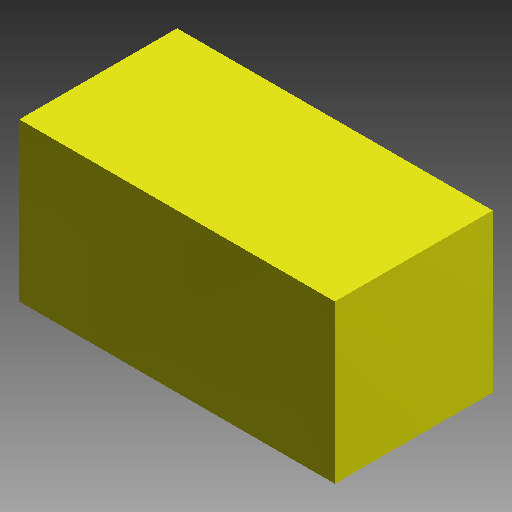
# Autodesk Inventor part: 1K
Saved by Autodesk Inventor 2018.2 (Build 222227000, 227)
## iProperties
Part Number: 1K
Material: Generic
Document SubType Name: Modeling
Designer: autocad
Appearance: R0603, 1K
Author: autocad
Autodesk Inventor part; units mm, degrees
ref_plane "YZ Plane" through (0, 0, 0) normal (1, 0, 0) x (0, 1, 0)
ref_plane "XZ Plane" through (0, 0, 0) normal (0, 1, 0) x (-1, 0, 0)
ref_plane "XY Plane" through (0, 0, 0) normal (0, 0, 1) x (1, 0, 0)
sketch "R0603, 1K_143" plane through (0, 0, 0) normal (0, 0, 1) x (1, 0, 0)
  line L0 (-0.7999, -0.3999) -> (-0.7999, 0.4001)
  line L1 (-0.7999, 0.4001) -> (0.8001, 0.4001)
  line L2 (0.8001, 0.4001) -> (0.8001, -0.3999)
  line L3 (0.8001, -0.3999) -> (-0.7999, -0.3999)
  constraints: 8 end point
extrude "Extrusion1" add sketch "R0603, 1K_143" along normal blind 0.8
body "Solid1"
